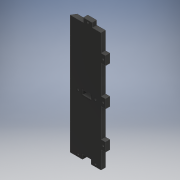
# Autodesk Inventor part: BA03
Saved by Autodesk Inventor 2017 (Build 210142000, 142)
## iProperties
Created: 2019-05-22
Part Number: BA03
Material: Wood (Cherry)
Document SubType Name: Modeling
Designer: Dell
Density: 0.63 g/cm^3
Appearance: Smooth - Black
Mass: 240.864 g
Surface Area: 748.675 cm^2
Volume: 382.323 cm^3
Author: Dell
Autodesk Inventor part; units mm, degrees
ref_plane "YZ Plane" through (0, 0, 0) normal (1, 0, 0) x (0, 1, 0)
ref_plane "XZ Plane" through (0, 0, 0) normal (0, 1, 0) x (-1, 0, 0)
ref_plane "XY Plane" through (0, 0, 0) normal (0, 0, 1) x (1, 0, 0)
sketch "Sketch1" plane through (0, 0, 0) normal (0, 0, 1) x (1, 0, 0)
  line L0 (0, 0) -> (88.9, 0)
  line L1 (88.9, 0) -> (88.9, 12.7)
  line L2 (88.9, 12.7) -> (7.3323, 12.7)
  line L3 (7.3323, 12.7) -> (0, 0)
  dimension "d0" = 88.9
  dimension "d1" = 12.7
  dimension "d2" = 60
  constraints: 8 end point, 2 perpendicular, 1 horizontal
  measures "d0" distance of L0.start L0.end
  measures "d1" distance of L0.end L1.end
  measures "d2" angle of L0 L3
extrude "Extrusion1" add sketch "Sketch1" along normal blind 342.9
sketch "Sketch2" plane through (0, 0, 0) normal (0, -1, 0) x (1, 0, 0)
  line L0 (38.1, 342.9) -> (63.5, 342.9)
  line L1 (63.5, 342.9) -> (63.5, 355.6)
  line L2 (63.5, 355.6) -> (38.1, 355.6)
  line L3 (38.1, 355.6) -> (38.1, 342.9)
  line L4 (0, 342.9) -> (101.6, 342.9)
  line L5 (0, 342.9) -> (88.9, 342.9) projected
  point P0 (0, 0)
  point P1 (50.8, 342.9)
  dimension "d5" = 25.4
  dimension "d6" = 12.7
  dimension "d9" = 101.6
  constraints: 10 end point, 2 midpoint, 2 parallel, 1 collinear, 1 horizontal, 1 perpendicular
  measures "d5" distance of L2.end L1.end
  measures "d6" distance of L1.end L0.end
  measures "d9" distance of L4.start L4.end
extrude "Extrusion2" add sketch "Sketch2" against normal blind 12.7
sketch "Sketch3" plane through (0, 0, 0) normal (0, -1, 0) x (1, 0, 0)
  line L0 (63.5, 342.9) -> (63.5, 355.6) projected
  line L1 (63.5, 355.6) -> (38.1, 355.6) projected
  circle A0 centre (50.8, 349.25) radius 2.25
  point P0 (0, 0)
  point P1 (50.8, 355.6)
  point P2 (63.5, 349.25)
  dimension "d10" = 4.5
  constraints: 2 midpoint, 1 centre point, 1 horizontal alignment, 1 vertical alignment
  measures "d10" diameter of A0
extrude "Extrusion3" cut sketch "Sketch3" against normal through all
sketch "Sketch4" plane through (0, 0, 0) normal (0, -1, 0) x (1, 0, 0)
  line L0 (88.9, 0) -> (88.9, 342.9) projected
  line L1 (88.9, 50.8) -> (101.6, 50.8)
  line L2 (101.6, 50.8) -> (101.6, 76.2)
  line L3 (101.6, 76.2) -> (88.9, 76.2)
  line L4 (88.9, 76.2) -> (88.9, 50.8)
  line L5 (88.9, 292.1) -> (101.6, 292.1)
  line L6 (101.6, 292.1) -> (101.6, 266.7)
  line L7 (101.6, 266.7) -> (88.9, 266.7)
  line L8 (88.9, 266.7) -> (88.9, 292.1)
  line L9 (88.9, 184.15) -> (101.6, 184.15)
  line L10 (101.6, 184.15) -> (101.6, 158.75)
  line L11 (101.6, 158.75) -> (88.9, 158.75)
  line L12 (88.9, 158.75) -> (88.9, 184.15)
  circle A0 centre (95.25, 279.4) radius 2.25
  circle A1 centre (95.25, 171.45) radius 2.25
  circle A2 centre (95.25, 63.5) radius 2.25
  point P0 (0, 0)
  point P1 (88.9, 171.45)
  point P2 (95.25, 292.1)
  point P3 (95.25, 184.15)
  point P4 (95.25, 76.2)
  point P5 (101.6, 279.4)
  point P6 (101.6, 171.45)
  point P7 (101.6, 63.5)
  dimension "d13" = 12.7
  dimension "d14" = 25.4
  dimension "d15" = 12.7
  dimension "d16" = 25.4
  dimension "d17" = 12.7
  dimension "d18" = 25.4
  dimension "d19" = 50.8
  dimension "d20" = 50.8
  dimension "d21" = 4.5
  dimension "d22" = 4.5
  dimension "d23" = 4.5
  constraints: 24 end point, 8 midpoint, 6 parallel, 3 centre point, 3 horizontal, 3 horizontal alignment, 3 perpendicular, 3 point on line, 3 vertical alignment
  measures "d13" distance of L3.end L2.end
  measures "d14" distance of L2.end L1.end
  measures "d15" distance of L6.end L7.end
  measures "d16" distance of L5.end L6.end
  measures "d17" distance of L10.end L11.end
  measures "d18" distance of L9.end L10.end
  measures "d19" distance from line of L0.end L5
  measures "d20" distance from line of L0.start L1
  measures "d21" diameter of A0
  measures "d22" diameter of A1
  measures "d23" diameter of A2
extrude "Extrusion4" add sketch "Sketch4" against normal blind 12.7
sketch "Sketch6" plane through (88.9, 0, 292.1) normal (0, 0, 1) x (1, 0, 0)
  line L0 (-88.9, 0) -> (-66.903, 12.7)
  line L1 (0, 12.7) -> (-81.5677, 12.7) projected
  line L2 (-88.9, 0) -> (0, 0) projected
  line L3 (-66.903, 12.7) -> (-66.903, 0)
  line L4 (-81.5677, 12.7) -> (-88.9, 0) projected
  line L5 (-77.9015, 6.35) -> (-77.9015, 12.7)
  line L6 (-77.9015, 12.7) -> (-81.5677, 12.7)
  dimension "d28" = 30
  dimension "d31" = 12.7
  constraints: 8 end point, 3 point on line, 1 collinear, 1 midpoint, 1 perpendicular, 1 vertical
  measures "d28" angle of L0 L2
  measures "d31" distance of L0.start L5.start
extrude "Extrusion6" cut sketch "Sketch6" against normal blind 25.4 contours L4 L1 L5 L0
sketch "Sketch7" plane through (88.9, 0, 184.15) normal (0, 0, 1) x (1, 0, 0)
  line L0 (-77.9015, 12.7) -> (-77.9015, 6.35) projected
  line L1 (-81.5677, 12.7) -> (-77.9015, 12.7) projected
  line L2 (-88.9, 0) -> (-81.5677, 12.7) projected
  line L3 (-77.9015, 6.35) -> (-88.9, 0) projected
  point P0 (-88.9, 0)
extrude "Extrusion7" cut sketch "Sketch7" against normal blind 25.4
sketch "Sketch8" plane through (88.9, 0, 76.2) normal (0, 0, 1) x (1, 0, 0)
  line L0 (-77.9015, 12.7) -> (-77.9015, 6.35) projected
  line L1 (-81.5677, 12.7) -> (-77.9015, 12.7) projected
  line L2 (-88.9, 0) -> (-81.5677, 12.7) projected
  line L3 (-77.9015, 6.35) -> (-88.9, 0) projected
  point P0 (-88.9, 0)
extrude "Extrusion8" cut sketch "Sketch8" against normal blind 25.4
sketch "Sketch10" plane through (7.3323, 12.7, 0) normal (0, 1, 0) x (1, 0, 0)
  circle A0 centre (15.7838, -6.35) radius 2.25
  line L0 (80.6319, -12.7) -> (0.9358, -12.7)
  circle A1 centre (65.7838, -6.35) radius 2.25
  line L1 (28.0838, -12.7) -> (53.4838, -12.7)
  line L2 (53.4838, -12.7) -> (53.4838, 0)
  line L3 (53.4838, 0) -> (28.0838, 0)
  line L4 (28.0838, 0) -> (28.0838, -12.7)
  line L5 (15.7838, -6.35) -> (65.7838, -6.35) construction
  line L6 (81.5677, 0) -> (0, 0) projected
  point P0 (-7.3323, 0)
  point P1 (40.7838, -6.35)
  point P2 (40.7838, -12.7)
  point P3 (40.7838, -12.7)
  point P4 (40.7838, 0)
  dimension "d39" = 4.5
  dimension "d40" = 6.35
  dimension "d41" = 4.5
  dimension "d42" = 25.4
  dimension "d43" = 12.7
  dimension "d44" = 50
  constraints: 12 end point, 7 midpoint, 3 horizontal, 2 centre point, 2 parallel, 1 perpendicular, 1 point on line, 1 vertical alignment
  measures "d39" diameter of A0
  measures "d40" distance from line of L0 L5.start
  measures "d41" diameter of A1
  measures "d42" distance of L3.end L2.end
  measures "d43" distance of L2.end L1.end
  measures "d44" distance of L5.start L5.end
extrude "Extrusion10" cut sketch "Sketch10" against normal through all
sketch "Sketch11" plane through (38.1, 0, 355.6) normal (0, -1, 0) x (1, 0, 0)
  line L0 (22.7162, -194.15) -> (-2.6838, -194.15)
  line L1 (-2.6838, -194.15) -> (-2.6838, -181.45)
  line L2 (-2.6838, -181.45) -> (22.7162, -181.45)
  line L3 (22.7162, -181.45) -> (22.7162, -194.15)
  line L4 (63.5, -171.45) -> (50.8, -171.45) projected
  line L5 (-2.6838, -342.9) -> (22.7162, -342.9) projected
  point P0 (-38.1, -355.6)
  point P1 (10.0162, -194.15)
  point P2 (10.0162, -342.9)
  dimension "d47" = 25.4
  dimension "d48" = 12.7
  dimension "d49" = 10
  constraints: 8 end point, 2 midpoint, 2 parallel, 1 horizontal, 1 perpendicular, 1 vertical alignment
  measures "d47" distance of L1.end L2.end
  measures "d48" distance of L0.end L1.end
  measures "d49" distance between parallel lines of L4 L2
extrude "Extrusion11" cut sketch "Sketch11" against normal through all
sketch "Sketch12" plane through (38.1, 0, 355.6) normal (0, -1, 0) x (1, 0, 0)
  circle A0 centre (-14.9838, -187.8) radius 2.25
  circle A1 centre (35.0162, -187.8) radius 2.25
  circle A2 centre (-14.9838, -349.25) radius 2.25 projected
  circle A3 centre (35.0162, -349.25) radius 2.25 projected
  line L0 (22.7162, -181.45) -> (22.7162, -194.15) projected
  point P0 (-38.1, -355.6)
  point P1 (22.7162, -187.8)
  dimension "d52" = 4.5
  dimension "d53" = 4.5
  constraints: 2 centre point, 2 horizontal alignment, 2 vertical alignment, 1 midpoint
  measures "d52" diameter of A0
  measures "d53" diameter of A1
extrude "Extrusion12" cut sketch "Sketch12" against normal through all contours A0 | A1
body "Solid1"
